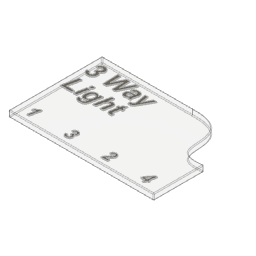
_ESP Lid.3ded5199-dcc8-4d53-9d14-e86b05d4e9f4 (Autodesk Fusion 360 design; units mm, degrees)
Autodesk Fusion 360 part; units mm, degrees
sketch "Sketch1" plane through (0, 0, 31) normal (0, 0, 1) x (-1, 0, 0)
  spline S0 degree 3 poles (-147.2811, 46.76) (-147.2863, 46.76) (-147.2914, 46.76) (-147.3016, 46.7598) (-147.3068, 46.7597) (-147.3119, 46.7595) knots -0.003077 -0.003077 -0.003077 -0.003077 -0.001538 -0.001538 0 0 0 0
  line L0 (-147.2811, 46.76) -> (-89.94, 46.76)
  line L1 (-89.94, 46.76) -> (-89.94, 105.64)
  line L2 (-89.94, 105.64) -> (-181.84, 105.64)
  line L3 (-181.84, 105.64) -> (-181.84, 74.5535)
  spline S1 degree 3 poles (-147.3119, 46.7595) (-148.1892, 46.7325) (-149.0681, 46.7246) (-151.5347, 46.7722) (-153.1205, 46.8816) (-155.9262, 47.313) (-157.1369, 47.5805) (-158.9414, 48.1641) (-159.5656, 48.4029) (-161.133, 49.1244) (-162.0548, 49.6766) (-163.3189, 50.6838) (-163.7241, 51.0545) (-164.7582, 52.1485) (-165.3283, 52.9373) (-166.0766, 54.321) (-166.3225, 54.8749) (-166.5314, 55.4366) (-167.0377, 56.798) (-167.3392, 58.2322) (-167.7974, 61.5711) (-167.8797, 63.4711) (-168.0363, 65.3647) (-168.1198, 66.3749) (-168.2247, 67.382) (-168.5218, 68.919) (-168.6544, 69.4635) (-168.8285, 69.9922) (-169.0848, 70.7701) (-169.4343, 71.5127) (-169.9339, 72.1637) (-170.3669, 72.7278) (-170.9089, 73.2002) (-172.2045, 73.9629) (-172.9658, 74.2413) (-174.5422, 74.6269) (-175.3713, 74.7382) (-177.1664, 74.861) (-178.1282, 74.8417) (-180.0045, 74.728) (-180.9225, 74.6399) (-181.84, 74.5535) knots 0.000761 0.000761 0.000761 0.000761 0.264079 0.264079 0.740333 0.740333 1.106683 1.106683 1.306501 1.306501 1.624187 1.624187 1.787585 1.787585 2.075226 2.075226 2.255002 2.255002 2.255002 2.690748 2.690748 3.260335 3.260335 3.260335 3.564218 3.564218 3.729968 3.729968 3.729968 3.973849 3.973849 3.973849 4.185188 4.185188 4.422884 4.422884 4.671815 4.671815 4.959442 4.959442 5.235791 5.235791 5.235791 5.235791
  line L4 (-97.0553, 109.8886) -> (-177.0949, 109.8886) construction
  line L5 (-177.0949, 109.8886) -> (-177.0949, 96.1122) construction
  line L6 (-177.0949, 96.1122) -> (-97.0553, 96.1122) construction
  line L7 (-97.0553, 96.1122) -> (-97.0553, 109.8886) construction
  line L8 (-92.5183, 65.3645) -> (-154.2843, 65.3645) construction
  line L9 (-154.2843, 65.3645) -> (-154.2843, 51.8597) construction
  line L10 (-154.2843, 51.8597) -> (-92.5183, 51.8597) construction
  line L11 (-92.5183, 51.8597) -> (-92.5183, 65.3645) construction
  line L12 (-92.6311, 77.1541) -> (-154.6263, 77.1541) construction
  line L13 (-154.6263, 77.1541) -> (-154.6263, 66.3715) construction
  line L14 (-154.6263, 66.3715) -> (-92.6311, 66.3715) construction
  line L15 (-92.6311, 66.3715) -> (-92.6311, 77.1541) construction
  line L16 (-100, 95) -> (-176, 95) construction
  line L17 (-176, 95) -> (-176, 87) construction
  line L18 (-176, 87) -> (-100, 87) construction
  line L19 (-100, 87) -> (-100, 95) construction
  dimension "d1" = 7
  dimension "d11" = 10
  dimension "d12" = 10
  dimension "d15" = 6
  text T0 "1       3       2       4" font "Arial" height 7 bold italic align left top in box 80.0396 x 13.7764 at (-97.0553, 109.8886) x (-1, 0) y (0, -1) spacing 1 kerned
  text T1 "3 Way" font "Arial" height 10 bold italic align left top in box 61.766 x 13.5048 at (-92.5183, 65.3645) x (-1, 0) y (0, -1) spacing 1 kerned
  text T2 "Light" font "Arial" height 10 bold italic align left top in box 61.9952 x 10.7827 at (-92.6311, 77.1541) x (-1, 0) y (0, -1) spacing 1 kerned
  constraint parallel L8 L14
  constraint parallel L1 L11
  constraint parallel L1 L7
sketch "sketch 10307" plane through (0, 0, 27) normal (0, 0, 1) x (-1, 0, 0)
  line L0 (-147.2888, 46.26) -> (-89.44, 46.26)
  line L1 (-89.44, 46.26) -> (-89.44, 106.14)
  line L2 (-89.44, 106.14) -> (-182.34, 106.14)
  line L3 (-182.34, 106.14) -> (-182.34, 74.0043)
  spline S0 degree 3 poles (-147.2888, 46.26) (-150.6096, 46.1574) (-153.7082, 46.3347) (-159.1015, 47.5278) (-160.782, 48.3635) (-163.103, 49.7634) (-164.2633, 50.7604) (-165.9986, 52.9987) (-166.8009, 54.401) (-168.2255, 59.3639) (-168.2987, 62.4706) (-168.66, 66.8403) (-168.8443, 68.4419) (-169.5239, 70.5051) (-169.8364, 71.2154) (-170.7326, 72.3831) (-171.2152, 72.811) (-172.4466, 73.5137) (-173.3583, 73.9081) (-177.2522, 74.516) (-179.3167, 74.2869) (-182.34, 74.0043) knots -14.954017 -14.954017 -14.954017 -14.954017 -13.094513 -13.094513 -11.321554 -11.321554 -9.035694 -9.035694 -7.073539 -7.073539 -4.267631 -4.267631 -2.775762 -2.775762 -2.059383 -2.059383 -1.476586 -1.476586 -0.910958 -0.910958 0 0 0 0
extrude "Extrude1" add sketch "sketch 10307" along normal blind 4 makes body 1 in component "ESP 4 Port Lid"
fillet "Fillet1" radius 0.5 1 edges at (135.89, -106.14, 31) 6 faces at (120.4067, -106.14, 28.3333) (108.7229, -66.22, 31) (182.34, -95.4281, 28.3333) (168.5396, -65.3838, 28.3333) (128.0059, -46.26, 28.3333) (89.44, -66.22, 28.3333) on bodies 1 in component "ESP 4 Port Lid"
extrude "Extrude2" [suppressed] in component "ESP 4 Port Lid"
extrude "Extrude3" [suppressed] in component "ESP 4 Port Lid"
extrude "Extrude4" [suppressed] in component "ESP 4 Port Lid"
extrude "Extrude5" [suppressed] in component "ESP 4 Port Lid"
extrude "Extrude6" [suppressed] in component "ESP 4 Port Lid"
extrude "Extrude1'" add sketch "Sketch1" along normal blind 0.5 separate body text T2 T1 T0 makes body 2 at (124.0257, -99.5323, 31) makes body 3 at (147.5148, -102.6952, 31) makes body 4 at (115.1576, -71.7726, 31) makes body 5 at (124.5775, -71.592, 31) makes body 6 at (103.5906, -67.5538, 31) makes body 7 at (103.411, -71.542, 31) makes body 8 at (111.8148, -72.1195, 31) makes body 9 at (94.1318, -72.481, 31) makes body 10 at (105.9221, -57.5259, 31) makes body 11 at (173.8499, -98.323, 31) makes body 12 at (99.7849, -99.1475, 31) makes body 13 at (97.057, -56.7455, 31) makes body 14 at (126.5633, -58.233, 31) makes body 15 at (122.9992, -57.776, 31) in component "ESP 4 Port Lid Letters"
other "Base Feature1''" in component "ESP Lid With Hook v2"
extrude "Extrude1''" [suppressed] in component "ESP Lid With Hook v2"
fillet "Fillet1'" [suppressed] in component "ESP Lid With Hook v2"
extrude "Extrude2'" [suppressed] in component "ESP Lid With Hook v2"
extrude "Extrude3'" [suppressed] in component "ESP Lid With Hook v2"
extrude "Extrude4'" [suppressed] in component "ESP Lid With Hook v2"
extrude "Extrude5'" [suppressed] in component "ESP Lid With Hook v2"
extrude "Extrude6'" [suppressed] in component "ESP Lid With Hook v2"
other "Base Feature1'''" in component "ESP Lid With Hook v2 (1)"
extrude "Extrude1'''" [suppressed] in component "ESP Lid With Hook v2 (1)"
fillet "Fillet1''" [suppressed] in component "ESP Lid With Hook v2 (1)"
extrude "Extrude2''" [suppressed] in component "ESP Lid With Hook v2 (1)"
extrude "Extrude3''" [suppressed] in component "ESP Lid With Hook v2 (1)"
extrude "Extrude4''" [suppressed] in component "ESP Lid With Hook v2 (1)"
extrude "Extrude5''" [suppressed] in component "ESP Lid With Hook v2 (1)"
extrude "Extrude6''" [suppressed] in component "ESP Lid With Hook v2 (1)"
combine "Combine1" [suppressed] in component "ESP Lid With Hook v2"
combine "Combine1'" [suppressed] in component "ESP Lid With Hook v2 (1)"
extrude "Extrude1''''" [suppressed] in component "4 Way Letters V2"
component "ESP 4 Port Lid" placed x (1, 0, 0) y (0, 1, 0) z (0, 0, 1) at (-0.0473, 0.0022, 0.0198)
component "ESP 4 Port Lid Letters" placed x (1, 0, 0) y (0, 1, 0) z (0, 0, 1) at (0, 0, 0)
